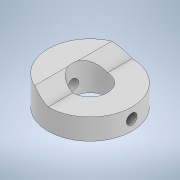
# Autodesk Inventor part: ang_wedge
Saved by Autodesk Inventor 2021 (Build 250183000, 183)
## iProperties
Created: 2024-02-29
Part Number: ang_wedge
Material: Generic
Document SubType Name: Modeling
Designer: Sebastián
Density: 1 g/cm^3
Appearance: Default
Author: Sebastián
Autodesk Inventor part; units mm, degrees
ref_plane "YZ Plane" through (0, 0, 0) normal (1, 0, 0) x (0, 1, 0)
ref_plane "XZ Plane" through (0, 0, 0) normal (0, 1, 0) x (-1, 0, 0)
ref_plane "XY Plane" through (0, 0, 0) normal (0, 0, 1) x (1, 0, 0)
sketch "Sketch1" plane through (0, 0, 0) normal (0, 1, 0) x (-1, 0, 0)
  circle A0 centre (0, 0) radius 10
  circle A1 centre (0, 0) radius 4.15
  dimension "d0" = 20
  dimension "d1" = 8.3
  constraints: 2 centre point, 2 coincident
  measures "d0" diameter of A0
  measures "d1" diameter of A1
extrude "Extrusion1" add sketch "Sketch1" along normal blind 5
sketch "Sketch2" plane through (0, 5, 0) normal (0, 1, 0) x (1, 0, 0)
  circle A0 centre (0, 0) radius 4.15 construction
  circle A1 centre (0, 0) radius 10 construction
  circle A2 centre (0, 0) radius 4.15 projected
  line L0 (0, -4.15) -> (0, -10)
  circle A3 centre (0, 0) radius 10 projected
  line L1 (0, 4.15) -> (0, 10)
  line L2 (14, 0) -> (-14, 0) construction
  arc A4 (0, 4.15) -> (0, -4.15) centre (0, 0) ccw construction
  arc A5 (0, 10) -> (0, -10) centre (0, 0) ccw
  arc A6 (0, 4.15) -> (0, -4.15) centre (0, 0) ccw
  line L3 (0, 0) -> (0, -10) construction
  point P0 (0, 4.15)
  dimension "d4" = 90
  constraints: 8 point on circle, 6 end point, 3 centre point, 3 coincident, 2 symmetric about line, 1 collinear, 1 vertical alignment, 3 other
  measures "d4" angle of L2 L3
extrude "Extrusion2" add sketch "Sketch2" along normal blind 2 contours A2 L0 A3 L1 picked at (-0.7977, -7.9531)
chamfer "Chamfer4" distance 4 distance2 2 1 edges at (0, 7, 7.075) measured on face at (-4.6768, 7, -6.482)
chamfer "Chamfer5" distance 4 distance2 2 1 edges at (0, 7, -7.075) measured on face at (-4.7092, 7, 6.0583)
sketch "Sketch3" plane through (0, 0, 0) normal (1, 0, 0) x (0, 1, 0)
  line L0 (5, 4.15) -> (5, -4.15) construction
  line L1 (5, -10) -> (5, 10) construction
  line L2 (0, -10) -> (0, 10) construction
  line L3 (-1.4, 0) -> (8.4, 0) construction
  circle A0 centre (2.5, 0) radius 1.25
  point P0 (0, 0)
  dimension "d22" = 2.5
  dimension "d23" = 2.5
  constraints: 1 centre point, 1 point on line
  measures "d22" diameter of A0
  measures "d23" distance from line of L0 A0.centre
extrude "Extrusion3" cut sketch "Sketch3" along normal through all both and the other way through all
body "Solid1"
